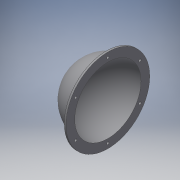
# Autodesk Inventor part: ROV Dome 4''
Saved by Autodesk Inventor 2016 (Build 200138000, 138)
## iProperties
Created: 2017-02-01
Part Number: ROV Dome 4''
Material: Generic
Document SubType Name: Modeling
Designer: Student
Density: 1 g/cm^3
Appearance: Default
Author: Student
Autodesk Inventor part; units mm, degrees
ref_plane "YZ Plane" through (0, 0, 0) normal (1, 0, 0) x (0, 1, 0)
ref_plane "XZ Plane" through (0, 0, 0) normal (0, 1, 0) x (-1, 0, 0)
ref_plane "XY Plane" through (0, 0, 0) normal (0, 0, 1) x (1, 0, 0)
sketch "Sketch1" plane through (0, 0, 0) normal (0, 1, 0) x (-1, 0, 0)
  arc A0 (50.8, 0) -> (1.2863, 50.7837) centre (0, 0) ccw
  line L0 (1.2863, 50.7837) -> (1.2863, 57.15)
  line L1 (-1.2537, 57.15) -> (-1.2537, 48.2437)
  arc A1 (48.26, 0) -> (-1.2537, 48.2437) centre (0, 0) ccw
  line L2 (1.2863, 57.15) -> (-1.2537, 57.15)
  line L3 (50.8, 0) -> (48.2557, 0)
  dimension "d0" = 50.8
  dimension "d5" = 2.54
  dimension "d19" = 57.15
  constraints: 8 end point, 4 point on circle, 2 centre point, 2 horizontal, 1 coincident, 1 point on line, 1 vertical
  measures "d0" distance of point (0, 0) L0.start
  measures "d5" radial gap between concentric circles of A0 A1
  measures "d19" vertical distance of point (0, 0) L1.start
revolve "Revolution1" add sketch "Sketch1" angle 360 about axis through (-50.8, 0, 0) along (1, 0, 0)
sketch "Sketch2" plane through (-1.2863, 0, 0) normal (-1, 0, 0) x (0, 0, 1)
  circle A0 centre (0, 53.975) radius 1.7526
  circle A1 centre (0, 0) radius 50.7837 projected
  circle A2 centre (-46.7437, 26.9875) radius 1.7526
  circle A3 centre (-46.7437, -26.9875) radius 1.7526
  circle A4 centre (0, -53.975) radius 1.7526
  circle A5 centre (46.7437, -26.9875) radius 1.7526
  circle A6 centre (46.7437, 26.9875) radius 1.7526
  dimension "d10" = 3.5052
  dimension "d12" = 53.975
  dimension "d15" = 360
  constraints: 6 centre point, 13 other
  measures "d10" diameter of A0
  measures "d12" distance of point (0, 0) A0.centre
extrude "Extrusion1" cut sketch "Sketch2" against normal blind 254 contours A0 | A2 | A3 | A4 | A5 | A6
body "Solid1"
